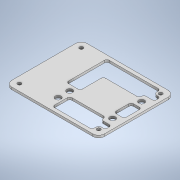
# Autodesk Inventor part: Trippeldekker_Øvre plate
Saved by Autodesk Inventor 2022 (Build 260153000, 153)
## iProperties
Created: 2021-08-17
Part Number: Trippeldekker_Øvre plate
Material: Generic
Document SubType Name: Modeling
Designer: Bruker
Density: 1 g/cm^3
Appearance: Default
Author: Bruker
Autodesk Inventor part; units mm, degrees
ref_plane "YZ Plane" through (0, 0, 0) normal (1, 0, 0) x (0, 1, 0)
ref_plane "XZ Plane" through (0, 0, 0) normal (0, 1, 0) x (-1, 0, 0)
ref_plane "XY Plane" through (0, 0, 0) normal (0, 0, 1) x (1, 0, 0)
sketch "Sketch1" plane through (0, 0, 0) normal (0, 1, 0) x (-1, 0, 0)
  line L0 (0, 0) -> (80, 0)
  line L1 (80, 0) -> (80, -65)
  line L2 (80, -65) -> (0, -65)
  line L3 (0, -65) -> (0, 0)
  dimension "d0" = 65
  dimension "d1" = 80
  constraints: 8 end point, 2 parallel, 1 horizontal, 1 perpendicular
  measures "d0" distance of L0.end L1.end
  measures "d1" distance of L1.end L2.end
extrude "Grunnflate" add sketch "Sketch1" along normal blind 2
sketch "Sketch3" plane through (0, 2, 0) normal (0, 1, 0) x (1, 0, 0)
  line L0 (-3, 3) -> (-77, 3)
  line L1 (-77, 3) -> (-77, 62)
  line L2 (-77, 62) -> (-3, 62)
  line L3 (-3, 62) -> (-3, 3)
  line L4 (-80, 65) -> (-80, 0) projected
  line L5 (0, 65) -> (-80, 65) projected
  line L6 (0, 0) -> (0, 65) projected
  line L7 (-80, 0) -> (0, 0) projected
  line L8 (-55, 3) -> (-3, 3)
  line L9 (-3, 3) -> (-3, 62)
  line L10 (-3, 62) -> (-55, 62)
  line L11 (-55, 62) -> (-55, 3)
  line L12 (-55, 3) -> (-43, 3)
  line L13 (-43, 3) -> (-43, 27)
  line L14 (-43, 27) -> (-55, 27)
  line L15 (-55, 27) -> (-55, 3)
  line L16 (-43, 18) -> (-12, 18)
  line L17 (-12, 18) -> (-12, 47)
  line L18 (-12, 47) -> (-43, 47)
  line L19 (-43, 47) -> (-43, 18)
  line L20 (-12, 25) -> (-3, 25)
  line L21 (-3, 25) -> (-3, 14)
  line L22 (-3, 14) -> (-12, 14)
  line L23 (-12, 14) -> (-12, 25)
  line L24 (-12, 40) -> (-3, 40)
  line L25 (-3, 40) -> (-3, 51)
  line L26 (-3, 51) -> (-12, 51)
  line L27 (-12, 51) -> (-12, 40)
  point P0 (-12, 18)
  point P1 (-3, 40)
  point P2 (-3, 25)
  dimension "d14" = 3
  dimension "d15" = 3
  dimension "d16" = 3
  dimension "d17" = 3
  dimension "d18" = 52
  dimension "d19" = 0
  dimension "d20" = 0
  dimension "d21" = 0
  dimension "d22" = 34
  dimension "d23" = 0
  dimension "d24" = 24
  dimension "d25" = 0
  dimension "d26" = 15
  dimension "d27" = 15
  dimension "d28" = 9
  dimension "d29" = 0
  dimension "d30" = 0
  dimension "d31" = 22
  dimension "d32" = 11
  dimension "d33" = 0
  dimension "d34" = 22
  dimension "d35" = 11
  constraints: 48 end point, 12 parallel, 6 horizontal, 6 perpendicular, 2 point on line
  measures "d14" distance between parallel lines of L4 L1
  measures "d15" distance between parallel lines of L5 L2
  measures "d16" distance between parallel lines of L6 L3
  measures "d17" distance between parallel lines of L7 L0
  measures "d18" distance of L9.end L10.end
  measures "d19" distance between parallel lines of L3 L9
  measures "d20" distance between parallel lines of L2 L10
  measures "d21" distance between parallel lines of L0 L8
  measures "d22" distance between parallel lines of L1 L13
  measures "d23" distance between parallel lines of L11 L15
  measures "d24" distance of L12.end L13.end
  measures "d25" distance between parallel lines of L0 L12
  measures "d26" distance between parallel lines of L0 L16
  measures "d27" distance between parallel lines of L10 L18
  measures "d28" distance between parallel lines of L3 L17
  measures "d29" distance between parallel lines of L17 L23
  measures "d30" distance between parallel lines of L9 L21
  measures "d31" distance between parallel lines of L8 L20
  measures "d32" distance between parallel lines of L0 L22
  measures "d33" distance between parallel lines of L9 L25
  measures "d34" distance between parallel lines of L2 L24
  measures "d35" distance between parallel lines of L10 L26
extrude "Hull" cut sketch "Sketch3" against normal blind 2 contours L0 L13 L16 L23 L22 L3 | L20 L17 L24 L3 | L11 L2 L3 L26 L27 L18 L19 L14
fillet "Fillet1" radius 2 2 edges at (-3, 1, -62) (-3, 1, -3)
fillet "Fillet3" radius 2 5 edges at (-43, 1, -3) (-3, 1, -14) (-12, 1, -14) (-12, 1, -18) (-43, 1, -18)
fillet "Fillet4" radius 2 7 edges at (-55, 1, -62) (-3, 1, -51) (-12, 1, -51) (-12, 1, -47) (-43, 1, -47) (-43, 1, -27) (-55, 1, -27)
fillet "Fillet5" radius 2 4 edges at (-12, 1, -40) (-3, 1, -40) (-3, 1, -25) (-12, 1, -25)
sketch "Knapper Layout" plane through (0, 2, 0) normal (0, 1, 0) x (1, 0, 0)
  line L0 (-77, 3) -> (-3, 3)
  line L1 (-3, 3) -> (-3, 62)
  line L2 (-3, 62) -> (-77, 62)
  line L3 (-77, 62) -> (-77, 3)
  line L4 (0, 65) -> (-80, 65) projected
  line L5 (0, 0) -> (0, 65) projected
  line L6 (-80, 0) -> (0, 0) projected
  line L7 (-80, 65) -> (-80, 0) projected
  line L8 (-11, 17) -> (-5, 17)
  line L9 (-5, 17) -> (-5, 23)
  line L10 (-5, 23) -> (-11, 23)
  line L11 (-11, 23) -> (-11, 17)
  line L12 (-11, 42) -> (-5, 42)
  line L13 (-5, 42) -> (-5, 48)
  line L14 (-5, 48) -> (-11, 48)
  line L15 (-11, 48) -> (-11, 42)
  line L16 (-50, 9) -> (-44, 9)
  line L17 (-44, 9) -> (-44, 15)
  line L18 (-44, 15) -> (-50, 15)
  line L19 (-50, 15) -> (-50, 9)
  line L20 (-50, 19) -> (-44, 19)
  line L21 (-44, 19) -> (-44, 25)
  line L22 (-44, 25) -> (-50, 25)
  line L23 (-50, 25) -> (-50, 19)
  circle A0 centre (-47, 12) radius 2.5
  circle A1 centre (-47, 22) radius 2.5
  circle A2 centre (-8, 45) radius 2.5
  circle A3 centre (-8, 20) radius 2.5
  point P0 (-2, 65)
  point P1 (-78, 65)
  point P2 (0, 2)
  point P3 (0, 63)
  point P4 (-78, 0)
  point P5 (-2, 0)
  point P6 (-80, 63)
  point P7 (-80, 2)
  dimension "d45" = 3
  dimension "d46" = 3
  dimension "d47" = 3
  dimension "d48" = 3
  dimension "d49" = 20
  dimension "d50" = 14
  dimension "d51" = 20
  dimension "d52" = 14
  dimension "d53" = 8
  dimension "d54" = 8
  dimension "d55" = 2
  dimension "d56" = 2
  dimension "d57" = 33
  dimension "d58" = 33
  dimension "d59" = 6
  dimension "d60" = 6
  dimension "d61" = 4
  dimension "d62" = 6
  dimension "d63" = 6
  dimension "d64" = 6
  dimension "d65" = 5
  dimension "d67" = 5
  dimension "d68" = 5
  dimension "d69" = 5
  constraints: 40 end point, 10 parallel, 5 horizontal, 5 perpendicular, 4 centre point
  measures "d45" distance between parallel lines of L4 L2
  measures "d46" distance between parallel lines of L5 L1
  measures "d47" distance between parallel lines of L6 L0
  measures "d48" distance between parallel lines of L7 L3
  measures "d49" distance between parallel lines of L0 L10
  measures "d50" distance between parallel lines of L2 L14
  measures "d51" distance between parallel lines of L2 L12
  measures "d52" distance between parallel lines of L0 L8
  measures "d53" distance between parallel lines of L1 L11
  measures "d54" distance between parallel lines of L1 L15
  measures "d55" distance between parallel lines of L1 L13
  measures "d56" distance between parallel lines of L1 L9
  measures "d57" distance between parallel lines of L21 L3
  measures "d58" distance between parallel lines of L3 L17
  measures "d59" distance of L21.end L22.end
  measures "d60" distance of L17.end L18.end
  measures "d61" distance between parallel lines of L20 L18
  measures "d62" distance of L18.end L16.start
  measures "d63" distance of L22.end L20.start
  measures "d64" distance between parallel lines of L0 L16
  measures "d65" diameter of A2
  measures "d67" diameter of A3
  measures "d68" diameter of A0
  measures "d69" diameter of A1
extrude "Knappehull" cut sketch "Knapper Layout" against normal blind 9.75 contours A0 | A1 | A2 | A3
sketch "Sketch8" plane through (0, 2, 0) normal (0, 1, 0) x (1, 0, 0)
  line L0 (-80, 65) -> (-80, 0) projected
  line L1 (0, 0) -> (-80, 0)
  line L2 (-80, 0) -> (-80, 65)
  line L3 (-80, 65) -> (0, 65)
  line L4 (0, 65) -> (0, 0)
  line L5 (-78.825, 1.175) -> (-1.175, 1.175)
  line L6 (-1.175, 1.175) -> (-1.175, 63.825)
  line L7 (-1.175, 63.825) -> (-78.825, 63.825)
  line L8 (-78.825, 63.825) -> (-78.825, 1.175)
  circle A0 centre (-5.8, 59.2) radius 1.575
  circle A1 centre (-5.8, 59.2) radius 3
  arc A2 (-3, 60) -> (-5, 62) centre (-5, 60) ccw projected
  circle A3 centre (-5.8, 5.8) radius 1.575
  circle A4 centre (-5.8, 5.8) radius 3
  arc A5 (-5, 3) -> (-3, 5) centre (-5, 5) ccw projected
  circle A6 centre (-74.2, 5.8) radius 1.575
  circle A7 centre (-74.2, 59.2) radius 1.575
  point P0 (-3.0321, 60.3571)
  point P1 (-4.6429, 61.9679)
  point P2 (-3.0321, 4.6429)
  point P3 (-4.6429, 3.0321)
  dimension "d80" = 77.65
  dimension "d81" = 4.625
  dimension "d82" = 4.625
  dimension "d83" = 3.15
  dimension "d84" = 6
  dimension "d85" = 4.625
  dimension "d86" = 4.625
  dimension "d87" = 3.15
  dimension "d88" = 6
  dimension "d89" = 3.15
  dimension "d90" = 3.15
  dimension "d91" = 4.625
  dimension "d92" = 4.625
  dimension "d93" = 4.625
  dimension "d94" = 4.625
  constraints: 16 end point, 8 point on circle, 6 centre point, 4 parallel, 2 coincident, 2 perpendicular, 1 horizontal, 3 other
  measures "d80" distance of L6.end L7.end
  measures "d81" distance from line of L7 A0.centre
  measures "d82" distance from line of L6 A0.centre
  measures "d83" diameter of A0
  measures "d84" diameter of A1
  measures "d85" distance from line of L6 A3.centre
  measures "d86" distance from line of L5 A3.centre
  measures "d87" diameter of A3
  measures "d88" diameter of A4
  measures "d89" diameter of A7
  measures "d90" diameter of A6
  measures "d91" distance from line of L5 A6.centre
  measures "d92" distance from line of L8 A6.centre
  measures "d93" distance from line of L7 A7.centre
  measures "d94" distance from line of L8 A7.centre
extrude "Extrusion7" cut sketch "Sketch8" against normal blind 10 contours A6 | A7
extrude "Extrusion8" add sketch "Sketch8" against normal blind 2 contours A1 | A1 A2 | A4 | A4 A5
fillet "Fillet8" radius 2 4 edges at (-3, 1, -58.123) (-3, 1, -6.877) (-6.877, 1, -3) (-6.877, 1, -62)
fillet "Fillet9" radius 5 4 edges at (-80, 1, 0) (0, 1, 0) (0, 1, -65) (-80, 1, -65)
body "Solid1"
